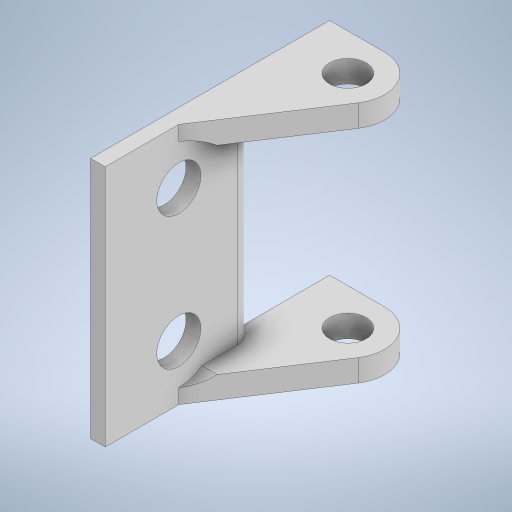
# Autodesk Inventor part: IdlerPulley Holder
Saved by Autodesk Inventor 2023 (Build 270158000, 158)
## iProperties
Created: 2023-04-27
Part Number: IdlerPulley Holder
Material: Generic
Document SubType Name: Modeling
Designer: ethan
Density: 1 g/cm^3
Appearance: Default
Author: ethan
Autodesk Inventor part; units mm, degrees
ref_plane "YZ Plane" through (0, 0, 0) normal (1, 0, 0) x (0, 1, 0)
ref_plane "XZ Plane" through (0, 0, 0) normal (0, 1, 0) x (-1, 0, 0)
ref_plane "XY Plane" through (0, 0, 0) normal (0, 0, 1) x (1, 0, 0)
sketch "Sketch1" plane through (0, 0, 0) normal (0, 1, 0) x (-1, 0, 0)
  line L0 (0, 0) -> (-20, 0) construction
  line L1 (-20, 0) -> (-20, -20) construction
  line L2 (-20, -20) -> (0, -20) construction
  line L3 (0, -20) -> (0, 0) construction
  circle A0 centre (-27.5, -27.5) radius 2.5
  circle A1 centre (-27.5, -27.5) radius 9 construction
  line L4 (-20, 0) -> (-22, 0)
  line L5 (-22, 0) -> (-22, -20)
  line L6 (-22, -20) -> (-20, -20)
  line L7 (-20, -20) -> (-20, 0)
  arc A2 (-27.5, -22.5) -> (-27.5, -32.5) centre (-27.5, -27.5) ccw
  line L8 (-27.5, -32.5) -> (-20.0167, -32.5)
  line L9 (-20, -20) -> (-20.0167, -32.5)
  line L10 (-22, -20) -> (-22, -20)
  arc A3 (-27.5, -32.5) -> (-27.5, -22.5) centre (-27.5, -27.5) ccw construction
  line L11 (-29.3102, -22.8392) -> (-22, -20)
  circle A4 centre (-27.5, -27.5) radius 11
  line L12 (-31.6807, -24.7575) -> (-22, -10)
  point P0 (-20.0167, -32.5)
  point P1 (-20, -19.4533)
  dimension "d12" = 18
  dimension "d17" = 0
  dimension "d0" = 20
  dimension "d1" = 20
  dimension "d4" = 5
  dimension "d11" = 7.5
  dimension "d14" = 7.5
  dimension "d15" = 2
  dimension "d16" = 10
  dimension "d34" = 2
  dimension "d36" = 10
  constraints: 27 end point, 6 point on circle, 4 centre point, 4 horizontal, 4 parallel, 3 coincident, 3 tangent, 2 perpendicular, 2 point on line, 1 midpoint, 8 other
  measures "d0" distance of L2.end L1.end
  measures "d1" distance of L1.end L0.end
  measures "d4" diameter of A0
  measures "d11" horizontal distance of L1.end A0.centre
  measures "d14" horizontal distance of A4.centre L1.end
  measures "d15" distance of L1.end L5.end
  measures "d16" diameter of A2
  measures "d36" distance from line of L4 L12.end
extrude "Extrusion1" add sketch "Sketch1" along normal mid plane 33 contours L7 A4 L5 L4 | L7 L6 L5 A4 | L9 L8 A2 L11 L6
extrude "Extrusion4" cut sketch "Sketch1" along normal mid plane 27 contours L9 L8 A2 L11 L6
sketch "Sketch3" plane through (22, -16.5, 0) normal (1, 0, 0) x (0, 0, -1)
  line L0 (20, 33) -> (0, 33) construction
  line L1 (10, 33) -> (10, -2) construction
  circle A0 centre (10, 25.5) radius 3
  circle A1 centre (10, 7.5) radius 3
  circle A2 centre (10, 25.5) radius 5.5
  circle A3 centre (10, 7.5) radius 5.5
  line L2 (20, 0) -> (0, 0) projected
  point P0 (16.4634, 0)
  dimension "d22" = 6
  dimension "d23" = 6
  dimension "d24" = 7.5
  dimension "d41" = 11
  dimension "d42" = 11
  dimension "d43" = 7.5
  constraints: 4 centre point, 2 coincident, 2 end point, 2 point on line, 1 midpoint, 1 vertical, 1 other
  measures "d22" diameter of A0
  measures "d23" diameter of A1
  measures "d24" distance from line of L0 A0.centre
  measures "d41" diameter of A2
  measures "d42" diameter of A3
extrude "Extrusion3" cut sketch "Sketch3" against normal up to surface (2 mm away) contours A0 | A1
extrude "Extrusion5" add sketch "Sketch1" along normal mid plane 33 contours L5 A4 L12 | L5 L11 A2 L12 A4
extrude "Extrusion6" cut sketch "Sketch1" along normal mid plane 27 contours L5 A4 L12 | L5 L11 A2 L12 A4
extrude "Extrusion7" cut sketch "Sketch3" along normal up to next
fillet "Fillet3" radius 2 1 edges at (22, 0, -20)
body "Solid1"
